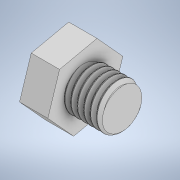
# Autodesk Inventor part: 1aThreads5_8x11ExternalBolt-V01
Saved by Autodesk Inventor 2021.1 (Build 251245010, 245A)
## iProperties
Created: 2020-10-17
Part Number: 1aThreads5_8x11ExternalBolt-V01
Material: Generic
Document SubType Name: Modeling
Designer: robst
Density: 1 g/cm^3
Appearance: Default
Author: robst
Autodesk Inventor part; units mm, degrees
ref_plane "YZ Plane" through (0, 0, 0) normal (1, 0, 0) x (0, 1, 0)
ref_plane "XZ Plane" through (0, 0, 0) normal (0, 1, 0) x (-1, 0, 0)
ref_plane "XY Plane" through (0, 0, 0) normal (0, 0, 1) x (1, 0, 0)
sketch "1aExternalThreadSketch" plane through (0, 0, 0) normal (0, 0, 1) x (1, 0, 0)
  line L0 (0, 6.2624) -> (0.8552, 7.7436)
  line L1 (1.056, 7.7436) -> (1.8453, 6.3767)
  arc A0 (1.8453, 6.3767) -> (2.2412, 6.3767) centre (2.0432, 6.491) ccw
  arc A1 (1.056, 7.7436) -> (0.8552, 7.7436) centre (0.9556, 7.6857) ccw
  line L2 (0, 7.8016) -> (20.6866, 7.8016) construction
  line L3 (0, 6.2624) -> (22.0033, 6.2624) construction
  line L4 (2.2412, 6.3767) -> (3.0304, 7.7436)
  line L5 (3.2312, 7.7436) -> (4.0205, 6.3767)
  arc A2 (3.2312, 7.7436) -> (3.0304, 7.7436) centre (3.1308, 7.6857) ccw
  line L6 (0, 6.2624) -> (0, 7.8016) construction
  line L7 (0.9556, 7.8016) -> (3.1308, 7.8016)
  line L8 (0, 0) -> (-12.7, 0)
  line L9 (-12.7, 0) -> (-12.7, 7.8016)
  line L10 (-12.7, 7.8016) -> (0, 7.8016)
  line L11 (0, 7.8016) -> (0, 0)
  line L12 (-19.6407, 0) -> (28.944, 0) projected
  dimension "d99" = 0.2286
  dimension "d102" = 60
  dimension "d105" = 6.2624
  dimension "d106" = 7.8016
  dimension "d108" = 60
  dimension "d111" = 0
  dimension "d112" = 60
  dimension "d129" = 7.8016
  dimension "d130" = 12.7
  constraints: 24 end point, 9 tangent, 8 point on circle, 3 centre point, 3 horizontal, 2 parallel, 2 perpendicular, 1 equal radius, 1 point on line
  measures "d99" radius of A0
  measures "d102" angle of L1 L0
  measures "d105" distance from line of L3 L8.start
  measures "d106" distance from line of L8.start L2
  measures "d108" angle of L5 L4
  measures "d111" distance from line of L6 L8.start
  measures "d112" angle of L4 L1
  measures "d129" distance between parallel lines of L8 L10
  measures "d130" distance between parallel lines of L9 L11
revolve "Revolution2" add sketch "1aExternalThreadSketch" angle 360 about axis through (-10, 0, 0) along (1, 0, 0) contours L8 L9 L10 L11
coil "Coil4" sketch "1aExternalThreadSketch" operation cut axis through (-10, 0, 0) along (-1, 0, 0) pitch 2.3091 turns 7.5 hand right contours A1 L7 A2 L4 A0 L1
sketch "Sketch9" plane through (-12.7, -2.8925, 4.3791) normal (-1, 0, 0) x (0, 0.3050259, 0.9523441)
  line L0 (8.6181, 10.9645) -> (8.6181, -2.7837)
  line L1 (8.6181, -2.7837) -> (-3.2881, -9.6577)
  line L2 (-3.2881, -9.6577) -> (-15.1944, -2.7837)
  line L3 (-15.1944, -2.7837) -> (-15.1944, 10.9645)
  line L4 (-15.1944, 10.9645) -> (-3.2881, 17.8386)
  line L5 (-3.2881, 17.8386) -> (8.6181, 10.9645)
  point P0 (-3.2881, 4.0904)
  point P1 (-3.2881, 4.0904)
  dimension "d148" = 23.8125
  constraints: 12 end point, 1 coincident, 1 vertical, 13 other
  measures "d148" distance between parallel lines of L0 L3
extrude "Extrusion5" add sketch "Sketch9" along normal blind 10.16
equation "\"d99\" = a1RootRadius"
equation "\"d102\" = threadAngle"
equation "\"d105\" = a1MinorRadius"
equation "\"d106\" = a1MajorRadius"
equation "\"d108\" = threadAngle"
equation "\"d112\" = threadAngle"
equation "\"d129\" = a1MajorRadius"
equation "\"d140\" = pitch"
equation "\"threadAngle\" = 60deg"
equation "\"a1MajorDiameter\" = 15.60322"
equation "\"a1MajorRadius\" = 0.5 * a1MajorDiameter"
equation "\"a1MinorDiameter\" = 12.52474"
equation "\"a1MinorRadius\" = 0.5 * a1MinorDiameter"
equation "\"a1RootRadius\" = 0.2286"
equation "\"a1CrestRadiusMax\" = 0.24892"
equation "\"pitch\" = 2.309091"
body "Solid4"
